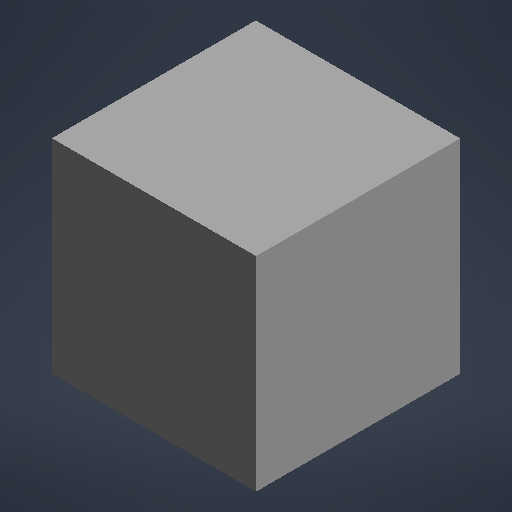
# Autodesk Inventor part: test_cube_10x10x10
Saved by Autodesk Inventor 2026 (Build 300175050, 175E)
## iProperties
Part Number: test_cube_10x10x10
Material: Generic
Document SubType Name: Modeling
Designer: Administrator
Appearance: Default
Author: Administrator
Autodesk Inventor part; units mm, degrees
ref_plane "YZ Plane" through (0, 0, 0) normal (1, 0, 0) x (0, 1, 0)
ref_plane "XZ Plane" through (0, 0, 0) normal (0, 1, 0) x (-1, 0, 0)
ref_plane "XY Plane" through (0, 0, 0) normal (0, 0, 1) x (1, 0, 0)
sketch "Sketch2" plane through (0, 0, 0) normal (0, 1, 0) x (-1, 0, 0)
  line L0 (0, 0) -> (10.0209, 0)
  line L1 (10.0209, 0) -> (10.0209, 10.0065)
  line L2 (10.0209, 10.0065) -> (0, 10.0065)
  line L3 (0, 10.0065) -> (0, 0)
  constraints: 8 end point, 2 parallel, 1 horizontal, 1 perpendicular
extrude "Extrusion2" add sketch "Sketch2" along normal blind 10
body "Solid2"
